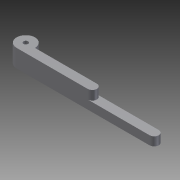
# Autodesk Inventor part: Traba
Saved by Autodesk Inventor 2011 (Build 150239000, 239)
## iProperties
Created: 2014-08-14
Part Number: Traba
Document SubType Name: Modeling
Designer: amatiasq
Density: 1 g/cm^3
Author: amatiasq
Autodesk Inventor part; units mm, degrees
ref_plane "YZ Plane" through (0, 0, 0) normal (1, 0, 0) x (0, 1, 0)
ref_plane "XZ Plane" through (0, 0, 0) normal (0, 1, 0) x (-1, 0, 0)
ref_plane "XY Plane" through (0, 0, 0) normal (0, 0, 1) x (1, 0, 0)
sketch "Boceto1" plane through (0, 0, 0) normal (0, 0, 1) x (1, 0, 0)
  line L0 (0, 0) -> (4, 0)
  line L1 (4, 0) -> (4, 4)
  line L2 (4, 4) -> (0, 4)
  line L3 (0, 4) -> (0, 0)
  line L4 (4, 0) -> (32, 0)
  line L5 (32, 0) -> (32, 2)
  line L6 (32, 2) -> (4, 2)
  line L7 (4, 2) -> (4, 0)
  dimension "d0" = 4
  dimension "d2" = 28
  dimension "d3" = 2
  dimension "d23" = 4
  constraints: 16 end point, 4 parallel, 2 horizontal, 2 perpendicular
  measures "d0" distance of L2.end L1.end
  measures "d2" distance of L6.end L5.end
  measures "d3" distance of L5.end L4.end
  measures "d23" distance of L2.end L0.start
extrude "Extrusión1" add sketch "Boceto1" along normal blind 1.9
fillet "Empalme8" radius 2 3 edges at (0, 0, 0.95) (0, 4, 0.95) (4, 4, 0.95)
fillet "Empalme9" radius 1 2 edges at (32, 2, 0.95) (32, 0, 0.95)
sketch "Boceto5" plane through (0, 0, 1.9) normal (0, 0, 1) x (1, 0, 0)
  arc A0 (4, 2) -> (2, 0) centre (2, 2) ccw projected
  point P0 (0, 0)
  constraints: 1 coincident
hole "Hole2" at (2, 2, 1.9) direction (0, 0, -1) diameter 1 end through all
sketch "Boceto6" plane through (0, 0, 1.9) normal (0, 0, 1) x (1, 0, 0)
  circle A0 centre (2, 2) radius 0.5 projected
  line L0 (4, 2) -> (31, 2) projected
  arc A1 (4, 2) -> (2, 0) centre (2, 2) ccw projected
  line L1 (31, 0) -> (2, 0) projected
  line L2 (18.5, 0) -> (18.5, 2)
  point P0 (0, 0)
  dimension "d34" = 14.5
  constraints: 2 end point, 2 point on line, 1 perpendicular
  measures "d34" distance from line of L2 L0.start
extrude "Extrusión3" add sketch "Boceto6" along normal blind 2
fillet "Empalme10" radius 1 2 edges at (18.5, 0, 2.9) (18.5, 2, 2.9)
